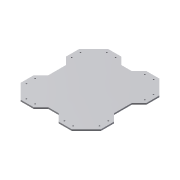
# Autodesk Inventor part: BackPlate
Saved by Autodesk Inventor 2014 (Build 180170000, 170)
## iProperties
Created: 2014-08-10
Part Number: BackPlate
Material: Generic
Document SubType Name: Modeling
Designer: Peele
Density: 1 g/cm^3
Appearance: White
Author: Peele
Autodesk Inventor part; units mm, degrees
ref_plane "YZ Plane" through (0, 0, 0) normal (1, 0, 0) x (0, 1, 0)
ref_plane "XZ Plane" through (0, 0, 0) normal (0, 1, 0) x (-1, 0, 0)
ref_plane "XY Plane" through (0, 0, 0) normal (0, 0, 1) x (1, 0, 0)
sketch "Sketch1" plane through (0, 0, 0) normal (0, 0, 1) x (1, 0, 0)
  line L0 (-112.5, -125) -> (112.5, -125)
  line L1 (112.5, -125) -> (112.5, 125)
  line L2 (112.5, 125) -> (-112.5, 125)
  line L3 (-112.5, 125) -> (-112.5, -125)
  line L4 (-112.5, -125) -> (112.5, 125) construction
  line L5 (112.5, -125) -> (-112.5, 125) construction
  point P0 (0, 0)
  dimension "d0" = 250
  dimension "d1" = 225
  constraints: 12 end point, 2 midpoint, 2 parallel, 1 horizontal, 1 perpendicular
  measures "d0" distance of L2.end L0.start
  measures "d1" distance of L1.end L2.end
extrude "Extrusion1" add sketch "Sketch1" along normal blind 5
sketch "Sketch2" plane through (0, 0, 5) normal (0, 0, 1) x (1, 0, 0)
  line L0 (112.5, -125) -> (112.5, 125) projected
  line L1 (112.5, 125) -> (-112.5, 125) projected
  line L2 (-112.5, 125) -> (-112.5, -125) projected
  line L3 (-112.5, 125) -> (-87.5, 150)
  line L4 (-87.5, 150) -> (-42.5, 150)
  line L5 (-42.5, 150) -> (-17.5, 125)
  line L6 (17.5, 125) -> (42.5, 150)
  line L7 (42.5, 150) -> (87.5, 150)
  line L8 (87.5, 150) -> (112.5, 125)
  line L9 (112.5, 125) -> (137.5, 100)
  line L10 (137.5, 100) -> (137.5, 55)
  line L11 (137.5, 55) -> (112.5, 30)
  line L12 (-112.5, 125) -> (-137.5, 100)
  line L13 (-137.5, 100) -> (-137.5, 55)
  line L14 (-137.5, 55) -> (-112.5, 30)
  line L15 (-17.5, 125) -> (-112.5, 30)
  line L16 (112.5, 30) -> (17.5, 125)
  circle A0 centre (-80, 137.5) radius 2.25
  circle A1 centre (-50, 137.5) radius 2.25
  circle A2 centre (50, 137.5) radius 2.25
  circle A3 centre (80, 137.5) radius 2.25
  circle A4 centre (125, 92.5) radius 2.25
  circle A5 centre (125, 62.5) radius 2.25
  circle A6 centre (-125, 92.5) radius 2.25
  circle A7 centre (-125, 62.5) radius 2.25
  point P0 (0, 0)
  dimension "d4" = 25
  dimension "d5" = 25
  dimension "d6" = 45
  dimension "d7" = 12.5
  dimension "d8" = 12.5
  dimension "d9" = 4.5
  dimension "d10" = 30
  dimension "d11" = 30
  dimension "d12" = 30
  dimension "d13" = 7.5
  dimension "d14" = 7.5
  dimension "d15" = 7.5
  dimension "d16" = 12.5
  constraints: 28 end point, 11 equal length, 8 centre point, 7 equal radius, 5 horizontal alignment, 4 perpendicular, 4 point on line, 2 collinear, 2 vertical alignment
  measures "d4" distance between parallel lines of L4 L1
  measures "d5" distance between parallel lines of L13 L2
  measures "d6" distance of L3.end L4.end
  measures "d7" distance from line of A0.centre L1
  measures "d8" distance from line of A6.centre L2
  measures "d9" diameter of A4
  measures "d10" distance of A3.centre A2.centre
  measures "d11" distance of A0.centre A1.centre
  measures "d12" distance of A5.centre A4.centre
  measures "d13" horizontal distance of A0.centre L3.end
  measures "d14" horizontal distance of L7.end A3.centre
  measures "d15" vertical distance of L9.end A4.centre
  measures "d16" distance from line of A4.centre L0
extrude "Extrusion2" add sketch "Sketch2" against normal blind 5 contours L0 L9 L10 L11 | L1 L6 L7 L8 | L1 L3 L4 L5 | L2 L14 L13 L12
mirror "Mirror1" about plane through (0, 0, 0) normal (0, 1, 0) of "Extrusion2"
equation "\"d8\" = d7"
equation "\"d11\" = d10"
equation "\"d12\" = d10"
equation "\"d13\" = -0.5 * d11 + 0.5 * d6"
equation "\"d14\" = d13"
equation "\"d15\" = d14"
body "Solid1"
